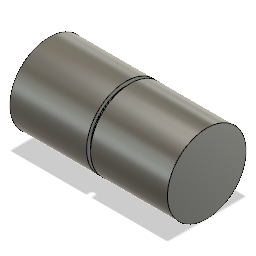
Table_17p1_Problem_15 (Autodesk Fusion 360 design; units mm, degrees)
Autodesk Fusion 360 part; units mm, degrees
sketch "Sketch1" plane through (0, 0, 0) normal (0, 0, 1) x (1, 0, 0)
  line L0 (100, 0) -> (100, 50)
  line L1 (100, 50) -> (2.5, 50)
  line L2 (2.5, 50) -> (2.5, 45)
  arc A0 (0, 42.5) -> (2.5, 45) centre (0, 45) ccw
  line L3 (0, 0) -> (100, 0) construction
  line L4 (0, 0) -> (0, 45) construction
  line L5 (0, 42.5) -> (100, 42.5) construction
  line L6 (100, 0) -> (100, -50) construction
  line L7 (100, -50) -> (2.5, -50) construction
  line L8 (2.5, -50) -> (2.5, -45) construction
  arc A1 (2.5, -45) -> (0, -42.5) centre (0, -45) ccw construction
  arc A2 (-2.5, 45) -> (0, 42.5) centre (0, 45) ccw
  line L9 (-2.5, 50) -> (-2.5, 45)
  line L10 (-100, 50) -> (-2.5, 50)
  line L11 (-100, 0) -> (-100, 50)
  line L12 (-100, 0) -> (-100, -50) construction
  line L13 (-100, -50) -> (-2.5, -50) construction
  line L14 (-2.5, -50) -> (-2.5, -45) construction
  arc A3 (0, -42.5) -> (-2.5, -45) centre (0, -45) ccw construction
  line L15 (100, 0) -> (-100, 0)
  dimension "Notch_Radius" = 2.5
  dimension "Notch_Height" = 7.5
  dimension "Bar_Diameter" = 100
  dimension "Bar_Length" = 200
  constraint vertical L0
  constraint perpendicular L0 L1
  constraint perpendicular L1 L2
  constraint tangent L2 A0
  constraint coincident L3.start L4.start
  constraint perpendicular L0 L3
  constraint coincident A0.centre L4.end
  constraint vertical L4
  constraint coincident A0.start L4
  constraint coincident L4 A0.start
  constraint coincident L0 L5.end
  constraint perpendicular L0 L5
  constraint tangent A0 L5
  constraint symmetric L0.start L3 L6.start
  constraint symmetric L0.end L3 L6.end
  constraint symmetric L1.end L3 L7.end
  constraint symmetric L2.end L3 L8.end
  constraint symmetric A0.start L3 A1.end
  constraint symmetric A0 L3 A1
  constraint symmetric L0.start L4 L11.start
  constraint symmetric L0.end L4 L10.start
  constraint symmetric L1.end L4 L9.start
  constraint symmetric L2.end L4 A2.start
  constraint symmetric A0.start L4 L5.start
  constraint symmetric A0 L4 A2
  constraint symmetric L4 L0.start L11.start
  constraint symmetric L4 L6.end L12.end
  constraint symmetric L4 L7.end L13.end
  constraint symmetric L4 L8.end L14.end
  constraint symmetric L4 A1.end A3.start
  constraint symmetric L4 A1 A3
  measures "Notch_Radius" radius of A0
  measures "Notch_Height" distance of L1 L5
  measures "Bar_Diameter" distance of L10 L13
  measures "Bar_Length" distance of L0 L11
revolve "Revolve1" add sketch "Sketch1" angle 360 about axis through (0, 0, 0) along (1, 0, 0)
